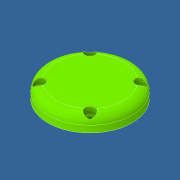
# Autodesk Inventor part: Cover_G2
Saved by Autodesk Inventor 2016 (Build 200138000, 138)
## iProperties
Created: 2015-09-10
Part Number: Cover_G2
Material: ABS-Kunststoff
Document SubType Name: Modeling
Designer: 4ndreas
Density: 1.06 g/cm^3
Appearance: Glatt - grün
Mass: 12.0516 g
Surface Area: 60.2207 cm^2
Volume: 11.3695 cm^3
Author: 4ndreas
Autodesk Inventor part; units mm, degrees
ref_plane "YZ Plane" through (0, 0, 0) normal (1, 0, 0) x (0, 1, 0)
ref_plane "XZ Plane" through (0, 0, 0) normal (0, 1, 0) x (-1, 0, 0)
ref_plane "XY Plane" through (0, 0, 0) normal (0, 0, 1) x (1, 0, 0)
sketch "Skizze1" plane through (0, 0, 0) normal (0, 0, 1) x (1, 0, 0)
  circle A0 centre (0, 0) radius 11.1 construction
  circle A1 centre (0, 0) radius 25 projected
  circle A2 centre (0, 0) radius 15
  circle A3 centre (-15, -15) radius 1.25 projected
  circle A4 centre (15, 15) radius 1.25 projected
  circle A5 centre (15, -15) radius 1.25 projected
  circle A6 centre (-15, 15) radius 1.25 projected
  point P0 (0, 0)
  dimension "d0" = 30
  constraints: 1 centre point, 1 coincident
  measures "d0" diameter of A2
extrude "Extrusion1" add sketch "Skizze1" along normal blind 9 contours A1 | A3 | A4 | A5 | A6
sketch "Skizze2" plane through (0, 0, 9) normal (0, 0, 1) x (1, 0, 0)
  circle A0 centre (0, 0) radius 15 projected
  circle A1 centre (0, 0) radius 25 projected
  point P0 (0, 0)
extrude "Extrusion2" add sketch "Skizze2" against normal blind 2 contours A0
fillet "Rundung1" radius 5 1 edges at (-25, 0, 9)
sketch "Skizze3" plane through (0, 0, 9) normal (0, 0, 1) x (1, 0, 0)
  line L0 (-15, -15) -> (15, -15)
  line L1 (15, -15) -> (15, 15)
  line L2 (15, 15) -> (-15, 15)
  line L3 (-15, 15) -> (-15, -15)
  line L4 (-15, -15) -> (15, 15) construction
  line L5 (15, -15) -> (-15, 15) construction
  point P0 (0, 0)
  dimension "d6" = 30
  constraints: 12 end point, 2 midpoint, 2 parallel, 2 perpendicular, 1 horizontal
  measures "d6" distance between parallel lines of L3 L1
hole "Bohrung1" at (-15, 15, 9) at (15, 15, 9) at (15, -15, 9) at (-15, -15, 9) direction (0, 0, -1) diameter 3 end through all counterbore diameter 6 counterbore depth 4
